Autodesk Fusion 360 part; units mm, degrees
note: some values were not read from the file. Set by a fixed rule: which sketch regions a step uses.
(part 47 of 59)
  spline S2 degree 5 poles (-27.3251, 22.3472) (-27.3252, 22.3472) (-27.3254, 22.3473) (-27.3257, 22.3474) (-27.3262, 22.3475) (-27.3269, 22.3478) (-27.3277, 22.3481) (-27.3286, 22.3484) (-27.3296, 22.3487) (-27.3308, 22.3491) (-27.332, 22.3495) (-27.3334, 22.35) (-27.3348, 22.3505) (-27.3364, 22.351) (-27.338, 22.3515) (-27.3398, 22.3521) (-27.3416, 22.3527) (-27.3435, 22.3533) (-27.3456, 22.3539) (-27.3477, 22.3546) (-27.3499, 22.3553) (-27.3523, 22.356) (-27.3547, 22.3568) (-27.3572, 22.3575) (-27.3598, 22.3583) (-27.3625, 22.3591) (-27.3652, 22.36) (-27.3681, 22.3608) (-27.371, 22.3617) (-27.3741, 22.3626) (-27.3772, 22.3635) (-27.3804, 22.3645) (-27.3837, 22.3654) (-27.387, 22.3664) (-27.3905, 22.3674) (-27.394, 22.3684) (-27.3976, 22.3694) (-27.4013, 22.3704) (-27.4051, 22.3715) (-27.409, 22.3725) (-27.4129, 22.3736) (-27.4169, 22.3747) (-27.421, 22.3758) (-27.4252, 22.3769) (-27.4294, 22.378) (-27.4337, 22.3792) (-27.4381, 22.3803) (-27.4426, 22.3815) (-27.4471, 22.3827) (-27.4517, 22.3838) (-27.4564, 22.385) (-27.4612, 22.3862) (-27.466, 22.3874) (-27.4709, 22.3887) (-27.4759, 22.3899) (-27.481, 22.3911) (-27.4861, 22.3924) (-27.4912, 22.3936) (-27.4965, 22.3949) (-27.5018, 22.3962) (-27.5072, 22.3974) (-27.5127, 22.3987) (-27.5182, 22.4) (-27.5238, 22.4013) (-27.5294, 22.4026) (-27.5352, 22.4039) (-27.5409, 22.4052) (-27.5468, 22.4065) (-27.5527, 22.4079) (-27.5587, 22.4092) (-27.5647, 22.4105) (-27.5709, 22.4118) (-27.577, 22.4132) (-27.5833, 22.4145) (-27.5896, 22.4158) (-27.5959, 22.4172) (-27.6023, 22.4185) (-27.6088, 22.4199) (-27.6154, 22.4212) (-27.622, 22.4225) (-27.6286, 22.4239) (-27.6353, 22.4252) (-27.6421, 22.4266) (-27.649, 22.4279) (-27.6559, 22.4293) (-27.6628, 22.4306) (-27.6698, 22.432) (-27.6769, 22.4333) (-27.6841, 22.4347) (-27.6912, 22.436) (-27.6985, 22.4374) (-27.7058, 22.4387) (-27.7132, 22.4401) (-27.7206, 22.4414) (-27.728, 22.4428) (-27.7356, 22.4441) (-27.7431, 22.4454) (-27.7508, 22.4468) (-27.7585, 22.4481) (-27.7662, 22.4494) (-27.774, 22.4508) (-27.7819, 22.4521) (-27.7898, 22.4534) (-27.7977, 22.4547) (-27.8057, 22.456) (-27.8138, 22.4573) (-27.8219, 22.4586) (-27.8301, 22.4599) (-27.8383, 22.4612) (-27.8466, 22.4625) (-27.8549, 22.4638) (-27.8633, 22.4651) (-27.8717, 22.4664) (-27.8802, 22.4676) (-27.8887, 22.4689) (-27.8973, 22.4701) (-27.9059, 22.4714) (-27.9146, 22.4726) (-27.9233, 22.4739) (-27.9321, 22.4751) (-27.9409, 22.4763) (-27.9498, 22.4776) (-27.9587, 22.4788) (-27.9677, 22.48) (-27.9767, 22.4812) (-27.9858, 22.4824) (-27.9949, 22.4836) (-28.004, 22.4847) (-28.0133, 22.4859) (-28.0225, 22.4871) (-28.0318, 22.4882) (-28.0412, 22.4894) (-28.0506, 22.4905) (-28.06, 22.4916) (-28.0695, 22.4928) (-28.079, 22.4939) (-28.0886, 22.495) (-28.0982, 22.4961) (-28.1079, 22.4972) (-28.1176, 22.4983) (-28.1274, 22.4993) (-28.1372, 22.5004) (-28.147, 22.5014) (-28.1569, 22.5025) (-28.1668, 22.5035) (-28.1768, 22.5045) (-28.1868, 22.5055) (-28.1969, 22.5065) (-28.207, 22.5075) (-28.2172, 22.5085) (-28.2274, 22.5095) (-28.2376, 22.5104) (-28.2479, 22.5114) (-28.2582, 22.5123) (-28.2686, 22.5133) (-28.279, 22.5142) (-28.2894, 22.5151) (-28.2999, 22.516) (-28.3105, 22.5169) (-28.321, 22.5177) (-28.3317, 22.5186) (-28.3423, 22.5195) (-28.353, 22.5203) (-28.3638, 22.5211) (-28.3745, 22.5219) (-28.3854, 22.5227) (-28.3962, 22.5235) (-28.4071, 22.5243) (-28.4181, 22.5251) (-28.429, 22.5258) (-28.44, 22.5266) (-28.4511, 22.5273) (-28.4622, 22.528) (-28.4733, 22.5287) (-28.4845, 22.5294) (-28.4957, 22.5301) (-28.507, 22.5308) (-28.5183, 22.5314) (-28.5296, 22.5321) (-28.541, 22.5327) (-28.5524, 22.5333) (-28.5638, 22.5339) (-28.5753, 22.5345) (-28.5868, 22.5351) (-28.5984, 22.5356) (-28.61, 22.5362) (-28.6216, 22.5367) (-28.6333, 22.5372) (-28.645, 22.5377) (-28.6567, 22.5382) (-28.6685, 22.5387) (-28.6803, 22.5392) (-28.6922, 22.5396) (-28.7041, 22.54) (-28.716, 22.5405) (-28.728, 22.5409) (-28.74, 22.5412) (-28.752, 22.5416) (-28.7641, 22.542) (-28.7762, 22.5423) (-28.7883, 22.5427) (-28.8005, 22.543) (-28.8127, 22.5433) (-28.8249, 22.5436) (-28.8372, 22.5438) (-28.8495, 22.5441) (-28.8619, 22.5443) (-28.8743, 22.5445) (-28.8867, 22.5448) (-28.8991, 22.5449) (-28.9116, 22.5451) (-28.9241, 22.5453) (-28.9367, 22.5454) (-28.9493, 22.5456) (-28.9619, 22.5457) (-28.9745, 22.5458) (-28.9872, 22.5458) (-29, 22.5459) (-29.0127, 22.546) (-29.0255, 22.546) (-29.0383, 22.546) (-29.0512, 22.546) (-29.0641, 22.546) (-29.077, 22.546) (-29.0899, 22.5459) (-29.1029, 22.5458) (-29.1159, 22.5458) (-29.129, 22.5457) (-29.142, 22.5455) (-29.1551, 22.5454) (-29.1683, 22.5453) (-29.1815, 22.5451) (-29.1947, 22.5449) (-29.2079, 22.5447) (-29.2212, 22.5445) (-29.2345, 22.5442) (-29.2478, 22.544) (-29.2612, 22.5437) (-29.2745, 22.5434) (-29.288, 22.5431) (-29.3014, 22.5428) (-29.3122, 22.5425) (-29.3203, 22.5423) (-29.3257, 22.5422) (-29.3284, 22.5421) knots 0 0 0 0 0 0 0.00416667 0.00833333 0.0125 0.01666667 0.02083333 0.025 0.02916667 0.03333333 0.0375 0.04166667 0.04583333 0.05 0.05416667 0.05833333 0.0625 0.06666667 0.07083333 0.075 0.07916667 0.08333333 0.0875 0.09166667 0.09583333 0.1 0.10416667 0.10833333 0.1125 0.11666667 0.12083333 0.125 0.12916667 0.13333333 0.1375 0.14166667 0.14583333 0.15 0.15416667 0.15833333 0.1625 0.16666667 0.17083333 0.175 0.17916667 0.18333333 0.1875 0.19166667 0.19583333 0.2 0.20416667 0.20833333 0.2125 0.21666667 0.22083333 0.225 0.22916667 0.23333333 0.2375 0.24166667 0.24583333 0.25 0.25416667 0.25833333 0.2625 0.26666667 0.27083333 0.275 0.27916667 0.28333333 0.2875 0.29166667 0.29583333 0.3 0.30416667 0.30833333 0.3125 0.31666667 0.32083333 0.325 0.32916667 0.33333333 0.3375 0.34166667 0.34583333 0.35 0.35416667 0.35833333 0.3625 0.36666667 0.37083333 0.375 0.37916667 0.38333333 0.3875 0.39166667 0.39583333 0.4 0.40416667 0.40833333 0.4125 0.41666667 0.42083333 0.425 0.42916667 0.43333333 0.4375 0.44166667 0.44583333 0.45 0.45416667 0.45833333 0.4625 0.46666667 0.47083333 0.475 0.47916667 0.48333333 0.4875 0.49166667 0.49583333 0.5 0.50416667 0.50833333 0.5125 0.51666667 0.52083333 0.525 0.52916667 0.53333333 0.5375 0.54166667 0.54583333 0.55 0.55416667 0.55833333 0.5625 0.56666667 0.57083333 0.575 0.57916667 0.58333333 0.5875 0.59166667 0.59583333 0.6 0.60416667 0.60833333 0.6125 0.61666667 0.62083333 0.625 0.62916667 0.63333333 0.6375 0.64166667 0.64583333 0.65 0.65416667 0.65833333 0.6625 0.66666667 0.67083333 0.675 0.67916667 0.68333333 0.6875 0.69166667 0.69583333 0.7 0.70416667 0.70833333 0.7125 0.71666667 0.72083333 0.725 0.72916667 0.73333333 0.7375 0.74166667 0.74583333 0.75 0.75416667 0.75833333 0.7625 0.76666667 0.77083333 0.775 0.77916667 0.78333333 0.7875 0.79166667 0.79583333 0.8 0.80416667 0.80833333 0.8125 0.81666667 0.82083333 0.825 0.82916667 0.83333333 0.8375 0.84166667 0.84583333 0.85 0.85416667 0.85833333 0.8625 0.86666667 0.87083333 0.875 0.87916667 0.88333333 0.8875 0.89166667 0.89583333 0.9 0.90416667 0.90833333 0.9125 0.91666667 0.92083333 0.925 0.92916667 0.93333333 0.9375 0.94166667 0.94583333 0.95 0.95416667 0.95833333 0.9625 0.96666667 0.97083333 0.975 0.97916667 0.98333333 0.9875 0.99166667 0.99583333 1 1 1 1 1 1
  arc A3 (-29.3284, 22.5421) -> (-29.6298, 21.6146) centre (0, 12.5) ccw
  spline S3 degree 5 poles (-29.6298, 21.6146) (-29.6276, 21.6129) (-29.6234, 21.6096) (-29.6169, 21.6047) (-29.6084, 21.5981) (-29.5977, 21.59) (-29.587, 21.5818) (-29.5763, 21.5737) (-29.5657, 21.5657) (-29.555, 21.5576) (-29.5444, 21.5496) (-29.5338, 21.5416) (-29.5232, 21.5337) (-29.5127, 21.5258) (-29.5021, 21.5179) (-29.4915, 21.5101) (-29.481, 21.5022) (-29.4705, 21.4945) (-29.46, 21.4867) (-29.4495, 21.479) (-29.4391, 21.4713) (-29.4286, 21.4637) (-29.4182, 21.456) (-29.4078, 21.4485) (-29.3974, 21.4409) (-29.387, 21.4334) (-29.3766, 21.4259) (-29.3663, 21.4184) (-29.356, 21.411) (-29.3457, 21.4036) (-29.3354, 21.3963) (-29.3251, 21.3889) (-29.3148, 21.3816) (-29.3046, 21.3744) (-29.2944, 21.3671) (-29.2842, 21.36) (-29.274, 21.3528) (-29.2638, 21.3457) (-29.2537, 21.3386) (-29.2435, 21.3315) (-29.2334, 21.3245) (-29.2233, 21.3175) (-29.2132, 21.3105) (-29.2032, 21.3036) (-29.1932, 21.2967) (-29.1831, 21.2898) (-29.1731, 21.283) (-29.1632, 21.2762) (-29.1532, 21.2694) (-29.1433, 21.2626) (-29.1334, 21.2559) (-29.1235, 21.2493) (-29.1136, 21.2426) (-29.1037, 21.236) (-29.0939, 21.2295) (-29.0841, 21.2229) (-29.0743, 21.2164) (-29.0646, 21.2099) (-29.0548, 21.2035) (-29.0451, 21.1971) (-29.0354, 21.1907) (-29.0257, 21.1844) (-29.016, 21.1781) (-29.0064, 21.1718) (-28.9968, 21.1656) (-28.9872, 21.1593) (-28.9776, 21.1532) (-28.9681, 21.147) (-28.9586, 21.1409) (-28.9491, 21.1348) (-28.9396, 21.1288) (-28.9302, 21.1228) (-28.9207, 21.1168) (-28.9113, 21.1109) (-28.902, 21.105) (-28.8926, 21.0991) (-28.8833, 21.0932) (-28.874, 21.0874) (-28.8647, 21.0817) (-28.8555, 21.0759) (-28.8462, 21.0702) (-28.837, 21.0645) (-28.8279, 21.0589) (-28.8187, 21.0533) (-28.8096, 21.0477) (-28.8005, 21.0422) (-28.7914, 21.0367) (-28.7824, 21.0312) (-28.7734, 21.0257) (-28.7644, 21.0203) (-28.7554, 21.015) (-28.7465, 21.0096) (-28.7376, 21.0043) (-28.7287, 20.999) (-28.7199, 20.9938) (-28.711, 20.9886) (-28.7022, 20.9834) (-28.6935, 20.9783) (-28.6847, 20.9732) (-28.676, 20.9681) (-28.6674, 20.963) (-28.6587, 20.958) (-28.6501, 20.9531) (-28.6415, 20.9481) (-28.633, 20.9432) (-28.6244, 20.9384) (-28.616, 20.9335) (-28.6075, 20.9287) (-28.5991, 20.9239) (-28.5907, 20.9192) (-28.5823, 20.9145) (-28.574, 20.9098) (-28.5657, 20.9052) (-28.5574, 20.9006) (-28.5491, 20.896) (-28.5409, 20.8915) (-28.5328, 20.887) (-28.5246, 20.8825) (-28.5165, 20.8781) (-28.5085, 20.8737) (-28.5004, 20.8693) (-28.4924, 20.865) (-28.4845, 20.8607) (-28.4765, 20.8565) (-28.4686, 20.8522) (-28.4608, 20.848) (-28.4529, 20.8439) (-28.4452, 20.8398) (-28.4374, 20.8357) (-28.4297, 20.8316) (-28.422, 20.8276) (-28.4144, 20.8236) (-28.4068, 20.8196) (-28.3992, 20.8157) (-28.3917, 20.8118) (-28.3842, 20.808) (-28.3767, 20.8042) (-28.3693, 20.8004) (-28.3619, 20.7966) (-28.3546, 20.7929) (-28.3473, 20.7892) (-28.3401, 20.7856) (-28.3329, 20.782) (-28.3257, 20.7784) (-28.3186, 20.7748) (-28.3115, 20.7713) (-28.3044, 20.7678) (-28.2974, 20.7644) (-28.2905, 20.761) (-28.2835, 20.7576) (-28.2767, 20.7543) (-28.2698, 20.751) (-28.263, 20.7477) (-28.2563, 20.7445) (-28.2496, 20.7412) (-28.2429, 20.7381) (-28.2363, 20.7349) (-28.2298, 20.7318) (-28.2233, 20.7288) (-28.2168, 20.7257) (-28.2104, 20.7227) (-28.204, 20.7198) (-28.1977, 20.7169) (-28.1914, 20.714) (-28.1851, 20.7111) (-28.179, 20.7083) (-28.1728, 20.7055) (-28.1667, 20.7027) (-28.1607, 20.7) (-28.1547, 20.6973) (-28.1488, 20.6947) (-28.1429, 20.692) (-28.1371, 20.6895) (-28.1313, 20.6869) (-28.1256, 20.6844) (-28.1199, 20.6819) (-28.1143, 20.6795) (-28.1087, 20.677) (-28.1032, 20.6747) (-28.0978, 20.6723) (-28.0924, 20.67) (-28.087, 20.6677) (-28.0818, 20.6655) (-28.0765, 20.6633) (-28.0714, 20.6611) (-28.0663, 20.659) (-28.0612, 20.6569) (-28.0562, 20.6548) (-28.0513, 20.6528) (-28.0464, 20.6508) (-28.0416, 20.6488) (-28.0369, 20.6469) (-28.0322, 20.645) (-28.0276, 20.6432) (-28.023, 20.6413) (-28.0185, 20.6395) (-28.0141, 20.6378) (-28.0097, 20.6361) (-28.0054, 20.6344) (-28.0012, 20.6327) (-27.997, 20.6311) (-27.9929, 20.6295) (-27.9889, 20.628) (-27.9849, 20.6265) (-27.9811, 20.625) (-27.9772, 20.6236) (-27.9735, 20.6222) (-27.9698, 20.6208) (-27.9662, 20.6194) (-27.9627, 20.6181) (-27.9593, 20.6169) (-27.9559, 20.6156) (-27.9526, 20.6144) (-27.9494, 20.6133) (-27.9462, 20.6121) (-27.9432, 20.6111) (-27.9402, 20.61) (-27.9373, 20.609) (-27.9345, 20.608) (-27.9318, 20.607) (-27.9291, 20.6061) (-27.9265, 20.6052) (-27.9241, 20.6044) (-27.9217, 20.6036) (-27.9194, 20.6028) (-27.9172, 20.602) (-27.915, 20.6013) (-27.913, 20.6007) (-27.9111, 20.6) (-27.9092, 20.5994) (-27.9075, 20.5988) (-27.9058, 20.5983) (-27.9043, 20.5978) (-27.9028, 20.5973) (-27.9015, 20.5969) (-27.9002, 20.5965) (-27.8991, 20.5962) (-27.898, 20.5958) (-27.8971, 20.5956) (-27.8963, 20.5953) (-27.8956, 20.5951) (-27.8951, 20.5949) (-27.8948, 20.5948) (-27.8946, 20.5948) (-27.8945, 20.5948) knots -1 -1 -1 -1 -1 -1 -0.99583333 -0.99166667 -0.9875 -0.98333333 -0.97916667 -0.975 -0.97083333 -0.96666667 -0.9625 -0.95833333 -0.95416667 -0.95 -0.94583333 -0.94166667 -0.9375 -0.93333333 -0.92916667 -0.925 -0.92083333 -0.91666667 -0.9125 -0.90833333 -0.90416667 -0.9 -0.89583333 -0.89166667 -0.8875 -0.88333333 -0.87916667 -0.875 -0.87083333 -0.86666667 -0.8625 -0.85833333 -0.85416667 -0.85 -0.84583333 -0.84166667 -0.8375 -0.83333333 -0.82916667 -0.825 -0.82083333 -0.81666667 -0.8125 -0.80833333 -0.80416667 -0.8 -0.79583333 -0.79166667 -0.7875 -0.78333333 -0.77916667 -0.775 -0.77083333 -0.76666667 -0.7625 -0.75833333 -0.75416667 -0.75 -0.74583333 -0.74166667 -0.7375 -0.73333333 -0.72916667 -0.725 -0.72083333 -0.71666667 -0.7125 -0.70833333 -0.70416667 -0.7 -0.69583333 -0.69166667 -0.6875 -0.68333333 -0.67916667 -0.675 -0.67083333 -0.66666667 -0.6625 -0.65833333 -0.65416667 -0.65 -0.64583333 -0.64166667 -0.6375 -0.63333333 -0.62916667 -0.625 -0.62083333 -0.61666667 -0.6125 -0.60833333 -0.60416667 -0.6 -0.59583333 -0.59166667 -0.5875 -0.58333333 -0.57916667 -0.575 -0.57083333 -0.56666667 -0.5625 -0.55833333 -0.55416667 -0.55 -0.54583333 -0.54166667 -0.5375 -0.53333333 -0.52916667 -0.525 -0.52083333 -0.51666667 -0.5125 -0.50833333 -0.50416667 -0.5 -0.49583333 -0.49166667 -0.4875 -0.48333333 -0.47916667 -0.475 -0.47083333 -0.46666667 -0.4625 -0.45833333 -0.45416667 -0.45 -0.44583333 -0.44166667 -0.4375 -0.43333333 -0.42916667 -0.425 -0.42083333 -0.41666667 -0.4125 -0.40833333 -0.40416667 -0.4 -0.39583333 -0.39166667 -0.3875 -0.38333333 -0.37916667 -0.375 -0.37083333 -0.36666667 -0.3625 -0.35833333 -0.35416667 -0.35 -0.34583333 -0.34166667 -0.3375 -0.33333333 -0.32916667 -0.325 -0.32083333 -0.31666667 -0.3125 -0.30833333 -0.30416667 -0.3 -0.29583333 -0.29166667 -0.2875 -0.28333333 -0.27916667 -0.275 -0.27083333 -0.26666667 -0.2625 -0.25833333 -0.25416667 -0.25 -0.24583333 -0.24166667 -0.2375 -0.23333333 -0.22916667 -0.225 -0.22083333 -0.21666667 -0.2125 -0.20833333 -0.20416667 -0.2 -0.19583333 -0.19166667 -0.1875 -0.18333333 -0.17916667 -0.175 -0.17083333 -0.16666667 -0.1625 -0.15833333 -0.15416667 -0.15 -0.14583333 -0.14166667 -0.1375 -0.13333333 -0.12916667 -0.125 -0.12083333 -0.11666667 -0.1125 -0.10833333 -0.10416667 -0.1 -0.09583333 -0.09166667 -0.0875 -0.08333333 -0.07916667 -0.075 -0.07083333 -0.06666667 -0.0625 -0.05833333 -0.05416667 -0.05 -0.04583333 -0.04166667 -0.0375 -0.03333333 -0.02916667 -0.025 -0.02083333 -0.01666667 -0.0125 -0.00833333 -0.00416667 0 0 0 0 0 0
  line L7 (-27.8945, 20.5948) -> (-27.8937, 20.5945)
  line L8 (-27.8937, 20.5945) -> (-27.6109, 20.5125)
  arc A4 (-27.6109, 20.5125) -> (-27.918, 19.3665) centre (0, 12.5) ccw
  line L9 (-27.918, 19.3665) -> (-28.2039, 19.4368)
  line L10 (-28.2039, 19.4368) -> (-28.2047, 19.437)
  spline S4 degree 5 poles (-28.2047, 19.437) (-28.2048, 19.437) (-28.205, 19.437) (-28.2053, 19.4371) (-28.2058, 19.4372) (-28.2065, 19.4374) (-28.2074, 19.4376) (-28.2083, 19.4378) (-28.2094, 19.4381) (-28.2106, 19.4383) (-28.2118, 19.4386) (-28.2132, 19.4389) (-28.2147, 19.4392) (-28.2163, 19.4396) (-28.218, 19.4399) (-28.2198, 19.4403) (-28.2217, 19.4407) (-28.2237, 19.4411) (-28.2258, 19.4416) (-28.228, 19.442) (-28.2303, 19.4425) (-28.2327, 19.4429) (-28.2351, 19.4434) (-28.2377, 19.4439) (-28.2404, 19.4445) (-28.2431, 19.445) (-28.246, 19.4455) (-28.2489, 19.4461) (-28.2519, 19.4466) (-28.255, 19.4472) (-28.2582, 19.4478) (-28.2615, 19.4484) (-28.2649, 19.449) (-28.2683, 19.4496) (-28.2719, 19.4502) (-28.2755, 19.4508) (-28.2792, 19.4515) (-28.283, 19.4521) (-28.2868, 19.4528) (-28.2908, 19.4534) (-28.2948, 19.4541) (-28.2989, 19.4547) (-28.3031, 19.4554) (-28.3074, 19.4561) (-28.3117, 19.4568) (-28.3161, 19.4574) (-28.3206, 19.4581) (-28.3252, 19.4588) (-28.3298, 19.4595) (-28.3345, 19.4602) (-28.3393, 19.4609) (-28.3442, 19.4616) (-28.3491, 19.4623) (-28.3541, 19.463) (-28.3592, 19.4637) (-28.3643, 19.4644) (-28.3695, 19.4651) (-28.3748, 19.4658) (-28.3802, 19.4665) (-28.3856, 19.4672) (-28.3911, 19.4679) (-28.3966, 19.4686) (-28.4023, 19.4693) (-28.408, 19.47) (-28.4137, 19.4707) (-28.4196, 19.4714) (-28.4255, 19.4721) (-28.4314, 19.4728) (-28.4374, 19.4735) (-28.4435, 19.4742) (-28.4497, 19.4749) (-28.4559, 19.4756) (-28.4622, 19.4763) (-28.4685, 19.4769) (-28.4749, 19.4776) (-28.4814, 19.4783) (-28.4879, 19.4789) (-28.4945, 19.4796) (-28.5011, 19.4803) (-28.5078, 19.4809) (-28.5146, 19.4816) (-28.5214, 19.4822) (-28.5283, 19.4828) (-28.5353, 19.4835) (-28.5423, 19.4841) (-28.5493, 19.4847) (-28.5564, 19.4853) (-28.5636, 19.4859) (-28.5709, 19.4865) (-28.5781, 19.4871) (-28.5855, 19.4877) (-28.5929, 19.4882) (-28.6004, 19.4888) (-28.6079, 19.4894) (-28.6154, 19.4899) (-28.6231, 19.4905) (-28.6307, 19.491) (-28.6385, 19.4915) (-28.6463, 19.4921) (-28.6541, 19.4926) (-28.662, 19.4931) (-28.67, 19.4936) (-28.678, 19.494) (-28.686, 19.4945) (-28.6941, 19.495) (-28.7023, 19.4954) (-28.7105, 19.4959) (-28.7187, 19.4963) (-28.727, 19.4968) (-28.7354, 19.4972) (-28.7438, 19.4976) (-28.7523, 19.498) (-28.7608, 19.4984) (-28.7694, 19.4987) (-28.778, 19.4991) (-28.7866, 19.4995) (-28.7953, 19.4998) (-28.8041, 19.5001) (-28.8129, 19.5005) (-28.8218, 19.5008) (-28.8307, 19.5011) (-28.8396, 19.5014) (-28.8486, 19.5016) (-28.8577, 19.5019) (-28.8668, 19.5021) (-28.8759, 19.5024) (-28.8851, 19.5026) (-28.8943, 19.5028) (-28.9036, 19.503) (-28.9129, 19.5032) (-28.9223, 19.5034) (-28.9317, 19.5036) (-28.9412, 19.5037) (-28.9507, 19.5038) (-28.9602, 19.504) (-28.9698, 19.5041) (-28.9795, 19.5042) (-28.9892, 19.5043) (-28.9989, 19.5043) (-29.0087, 19.5044) (-29.0185, 19.5044) (-29.0284, 19.5045) (-29.0383, 19.5045) (-29.0482, 19.5045) (-29.0582, 19.5045) (-29.0682, 19.5044) (-29.0783, 19.5044) (-29.0884, 19.5043) (-29.0986, 19.5043) (-29.1088, 19.5042) (-29.119, 19.5041) (-29.1293, 19.504) (-29.1396, 19.5038) (-29.15, 19.5037) (-29.1604, 19.5035) (-29.1708, 19.5034) (-29.1813, 19.5032) (-29.1919, 19.503) (-29.2024, 19.5028) (-29.213, 19.5025) (-29.2237, 19.5023) (-29.2344, 19.502) (-29.2451, 19.5017) (-29.2559, 19.5014) (-29.2667, 19.5011) (-29.2775, 19.5008) (-29.2884, 19.5004) (-29.2993, 19.5001) (-29.3103, 19.4997) (-29.3213, 19.4993) (-29.3323, 19.4989) (-29.3434, 19.4984) (-29.3545, 19.498) (-29.3657, 19.4975) (-29.3768, 19.497) (-29.3881, 19.4965) (-29.3993, 19.496) (-29.4106, 19.4955) (-29.422, 19.495) (-29.4333, 19.4944) (-29.4447, 19.4938) (-29.4562, 19.4932) (-29.4677, 19.4926) (-29.4792, 19.492) (-29.4907, 19.4913) (-29.5023, 19.4906) (-29.514, 19.49) (-29.5256, 19.4892) (-29.5373, 19.4885) (-29.549, 19.4878) (-29.5608, 19.487) (-29.5726, 19.4863) (-29.5844, 19.4855) (-29.5963, 19.4846) (-29.6082, 19.4838) (-29.6201, 19.483) (-29.6321, 19.4821) (-29.6441, 19.4812) (-29.6562, 19.4803) (-29.6682, 19.4794) (-29.6803, 19.4784) (-29.6925, 19.4775) (-29.7047, 19.4765) (-29.7169, 19.4755) (-29.7291, 19.4745) (-29.7414, 19.4735) (-29.7537, 19.4724) (-29.766, 19.4713) (-29.7784, 19.4702) (-29.7908, 19.4691) (-29.8032, 19.468) (-29.8157, 19.4669) (-29.8282, 19.4657) (-29.8407, 19.4645) (-29.8533, 19.4633) (-29.8659, 19.4621) (-29.8785, 19.4608) (-29.8912, 19.4596) (-29.9039, 19.4583) (-29.9166, 19.457) (-29.9293, 19.4556) (-29.9421, 19.4543) (-29.9549, 19.4529) (-29.9678, 19.4516) (-29.9806, 19.4501) (-29.9935, 19.4487) (-30.0065, 19.4473) (-30.0194, 19.4458) (-30.0324, 19.4443) (-30.0455, 19.4428) (-30.0585, 19.4413) (-30.0716, 19.4398) (-30.0847, 19.4382) (-30.0979, 19.4366) (-30.111, 19.435) (-30.1242, 19.4334) (-30.1375, 19.4317) (-30.1507, 19.4301) (-30.164, 19.4284) (-30.1773, 19.4267) (-30.1907, 19.425) (-30.2014, 19.4236) (-30.2094, 19.4225) (-30.2148, 19.4218) (-30.2174, 19.4214) knots 0 0 0 0 0 0 0.00416667 0.00833333 0.0125 0.01666667 0.02083333 0.025 0.02916667 0.03333333 0.0375 0.04166667 0.04583333 0.05 0.05416667 0.05833333 0.0625 0.06666667 0.07083333 0.075 0.07916667 0.08333333 0.0875 0.09166667 0.09583333 0.1 0.10416667 0.10833333 0.1125 0.11666667 0.12083333 0.125 0.12916667 0.13333333 0.1375 0.14166667 0.14583333 0.15 0.15416667 0.15833333 0.1625 0.16666667 0.17083333 0.175 0.17916667 0.18333333 0.1875 0.19166667 0.19583333 0.2 0.20416667 0.20833333 0.2125 0.21666667 0.22083333 0.225 0.22916667 0.23333333 0.2375 0.24166667 0.24583333 0.25 0.25416667 0.25833333 0.2625 0.26666667 0.27083333 0.275 0.27916667 0.28333333 0.2875 0.29166667 0.29583333 0.3 0.30416667 0.30833333 0.3125 0.31666667 0.32083333 0.325 0.32916667 0.33333333 0.3375 0.34166667 0.34583333 0.35 0.35416667 0.35833333 0.3625 0.36666667 0.37083333 0.375 0.37916667 0.38333333 0.3875 0.39166667 0.39583333 0.4 0.40416667 0.40833333 0.4125 0.41666667 0.42083333 0.425 0.42916667 0.43333333 0.4375 0.44166667 0.44583333 0.45 0.45416667 0.45833333 0.4625 0.46666667 0.47083333 0.475 0.47916667 0.48333333 0.4875 0.49166667 0.49583333 0.5 0.50416667 0.50833333 0.5125 0.51666667 0.52083333 0.525 0.52916667 0.53333333 0.5375 0.54166667 0.54583333 0.55 0.55416667 0.55833333 0.5625 0.56666667 0.57083333 0.575 0.57916667 0.58333333 0.5875 0.59166667 0.59583333 0.6 0.60416667 0.60833333 0.6125 0.61666667 0.62083333 0.625 0.62916667 0.63333333 0.6375 0.64166667 0.64583333 0.65 0.65416667 0.65833333 0.6625 0.66666667 0.67083333 0.675 0.67916667 0.68333333 0.6875 0.69166667 0.69583333 0.7 0.70416667 0.70833333 0.7125 0.71666667 0.72083333 0.725 0.72916667 0.73333333 0.7375 0.74166667 0.74583333 0.75 0.75416667 0.75833333 0.7625 0.76666667 0.77083333 0.775 0.77916667 0.78333333 0.7875 0.79166667 0.79583333 0.8 0.80416667 0.80833333 0.8125 0.81666667 0.82083333 0.825 0.82916667 0.83333333 0.8375 0.84166667 0.84583333 0.85 0.85416667 0.85833333 0.8625 0.86666667 0.87083333 0.875 0.87916667 0.88333333 0.8875 0.89166667 0.89583333 0.9 0.90416667 0.90833333 0.9125 0.91666667 0.92083333 0.925 0.92916667 0.93333333 0.9375 0.94166667 0.94583333 0.95 0.95416667 0.95833333 0.9625 0.96666667 0.97083333 0.975 0.97916667 0.98333333 0.9875 0.99166667 0.99583333 1 1 1 1 1 1
  arc A5 (-30.2174, 19.4214) -> (-30.4202, 18.4675) centre (0, 12.5) ccw
  spline S5 degree 5 poles (-30.4202, 18.4675) (-30.4179, 18.4661) (-30.4133, 18.4633) (-30.4064, 18.459) (-30.3972, 18.4534) (-30.3857, 18.4464) (-30.3742, 18.4394) (-30.3628, 18.4325) (-30.3513, 18.4255) (-30.3399, 18.4187) (-30.3285, 18.4118) (-30.3171, 18.405) (-30.3058, 18.3982) (-30.2944, 18.3914) (-30.2831, 18.3847) (-30.2718, 18.378) (-30.2605, 18.3713) (-30.2492, 18.3647) (-30.238, 18.3581) (-30.2268, 18.3515) (-30.2156, 18.3449) (-30.2044, 18.3384) (-30.1932, 18.3319) (-30.1821, 18.3255) (-30.1709, 18.3191) (-30.1598, 18.3127) (-30.1487, 18.3063) (-30.1377, 18.3) (-30.1266, 18.2937) (-30.1156, 18.2874) (-30.1046, 18.2811) (-30.0936, 18.2749) (-30.0826, 18.2688) (-30.0717, 18.2626) (-30.0608, 18.2565) (-30.0499, 18.2504) (-30.039, 18.2443) (-30.0281, 18.2383) (-30.0173, 18.2323) (-30.0065, 18.2263) (-29.9957, 18.2204) (-29.9849, 18.2145) (-29.9742, 18.2086) (-29.9634, 18.2028) (-29.9527, 18.197) (-29.9421, 18.1912) (-29.9314, 18.1854) (-29.9208, 18.1797) (-29.9102, 18.174) (-29.8996, 18.1683) (-29.889, 18.1627) (-29.8785, 18.1571) (-29.868, 18.1515) (-29.8575, 18.146) (-29.847, 18.1405) (-29.8366, 18.135) (-29.8262, 18.1296) (-29.8158, 18.1242) (-29.8054, 18.1188) (-29.7951, 18.1134) (-29.7847, 18.1081) (-29.7745, 18.1028) (-29.7642, 18.0975) (-29.754, 18.0923) (-29.7437, 18.0871) (-29.7336, 18.0819) (-29.7234, 18.0768) (-29.7133, 18.0717) (-29.7032, 18.0666) (-29.6931, 18.0615) (-29.683, 18.0565) (-29.673, 18.0515) (-29.663, 18.0466) (-29.653, 18.0416) (-29.6431, 18.0367) (-29.6332, 18.0319) (-29.6233, 18.027) (-29.6134, 18.0222) (-29.6036, 18.0175) (-29.5938, 18.0127) (-29.584, 18.008) (-29.5743, 18.0033) (-29.5646, 17.9987) (-29.5549, 17.994) (-29.5452, 17.9895) (-29.5356, 17.9849) (-29.526, 17.9804) (-29.5165, 17.9759) (-29.5069, 17.9714) (-29.4974, 17.967) (-29.4879, 17.9625) (-29.4785, 17.9582) (-29.4691, 17.9538) (-29.4597, 17.9495) (-29.4504, 17.9452) (-29.441, 17.941) (-29.4318, 17.9367) (-29.4225, 17.9325) (-29.4133, 17.9284) (-29.4041, 17.9242) (-29.395, 17.9201) (-29.3858, 17.9161) (-29.3767, 17.912) (-29.3677, 17.908) (-29.3587, 17.904) (-29.3497, 17.9001) (-29.3407, 17.8961) (-29.3318, 17.8922) (-29.3229, 17.8884) (-29.3141, 17.8846) (-29.3053, 17.8807) (-29.2965, 17.877) (-29.2878, 17.8732) (-29.279, 17.8695) (-29.2704, 17.8658) (-29.2617, 17.8622) (-29.2531, 17.8586) (-29.2446, 17.855) (-29.2361, 17.8514) (-29.2276, 17.8479) (-29.2191, 17.8444) (-29.2107, 17.8409) (-29.2023, 17.8375) (-29.194, 17.8341) (-29.1857, 17.8307) (-29.1775, 17.8273) (-29.1692, 17.824) (-29.1611, 17.8207) (-29.1529, 17.8175) (-29.1448, 17.8143) (-29.1368, 17.8111) (-29.1288, 17.8079) (-29.1208, 17.8047) (-29.1129, 17.8016) (-29.105, 17.7986) (-29.0971, 17.7955) (-29.0893, 17.7925) (-29.0815, 17.7895) (-29.0738, 17.7865) (-29.0661, 17.7836) (-29.0585, 17.7807) (-29.0509, 17.7778) (-29.0433, 17.775) (-29.0358, 17.7722) (-29.0284, 17.7694) (-29.021, 17.7666) (-29.0136, 17.7639) (-29.0063, 17.7612) (-28.999, 17.7586) (-28.9918, 17.7559) (-28.9846, 17.7533) (-28.9774, 17.7508) (-28.9703, 17.7482) (-28.9633, 17.7457) (-28.9563, 17.7432) (-28.9493, 17.7408) (-28.9424, 17.7383) (-28.9356, 17.7359) (-28.9288, 17.7336) (-28.922, 17.7312) (-28.9153, 17.7289) (-28.9087, 17.7266) (-28.9021, 17.7244) (-28.8955, 17.7222) (-28.889, 17.72) (-28.8826, 17.7178) (-28.8762, 17.7157) (-28.8699, 17.7136) (-28.8636, 17.7115) (-28.8573, 17.7094) (-28.8512, 17.7074) (-28.8451, 17.7054) (-28.839, 17.7035) (-28.833, 17.7015) (-28.827, 17.6996) (-28.8211, 17.6978) (-28.8153, 17.6959) (-28.8095, 17.6941) (-28.8038, 17.6923) (-28.7981, 17.6905) (-28.7925, 17.6888) (-28.7869, 17.6871) (-28.7815, 17.6854) (-28.776, 17.6838) (-28.7707, 17.6822) (-28.7654, 17.6806) (-28.7601, 17.679) (-28.7549, 17.6775) (-28.7498, 17.676) (-28.7448, 17.6745) (-28.7398, 17.673) (-28.7349, 17.6716) (-28.73, 17.6702) (-28.7252, 17.6689) (-28.7205, 17.6675) (-28.7158, 17.6662) (-28.7112, 17.6649) (-28.7067, 17.6637) (-28.7023, 17.6625) (-28.6979, 17.6613) (-28.6936, 17.6601) (-28.6893, 17.6589) (-28.6852, 17.6578) (-28.6811, 17.6567) (-28.6771, 17.6557) (-28.6731, 17.6546) (-28.6693, 17.6536) (-28.6655, 17.6527) (-28.6617, 17.6517) (-28.6581, 17.6508) (-28.6545, 17.6499) (-28.6511, 17.649) (-28.6477, 17.6481) (-28.6443, 17.6473) (-28.6411, 17.6465) (-28.6379, 17.6458) (-28.6349, 17.645) (-28.6319, 17.6443) (-28.629, 17.6436) (-28.6262, 17.643) (-28.6234, 17.6423) (-28.6208, 17.6417) (-28.6182, 17.6411) (-28.6158, 17.6406) (-28.6134, 17.64) (-28.6111, 17.6395) (-28.6089, 17.639) (-28.6069, 17.6386) (-28.6049, 17.6381) (-28.603, 17.6377) (-28.6012, 17.6374) (-28.5995, 17.637) (-28.5979, 17.6367) (-28.5964, 17.6363) (-28.595, 17.6361) (-28.5937, 17.6358) (-28.5925, 17.6356) (-28.5915, 17.6354) (-28.5905, 17.6352) (-28.5896, 17.635) (-28.5889, 17.6349) (-28.5884, 17.6348) (-28.5881, 17.6347) (-28.5879, 17.6347) (-28.5878, 17.6346) knots -1 -1 -1 -1 -1 -1 -0.99583333 -0.99166667 -0.9875 -0.98333333 -0.97916667 -0.975 -0.97083333 -0.96666667 -0.9625 -0.95833333 -0.95416667 -0.95 -0.94583333 -0.94166667 -0.9375 -0.93333333 -0.92916667 -0.925 -0.92083333 -0.91666667 -0.9125 -0.90833333 -0.90416667 -0.9 -0.89583333 -0.89166667 -0.8875 -0.88333333 -0.87916667 -0.875 -0.87083333 -0.86666667 -0.8625 -0.85833333 -0.85416667 -0.85 -0.84583333 -0.84166667 -0.8375 -0.83333333 -0.82916667 -0.825 -0.82083333 -0.81666667 -0.8125 -0.80833333 -0.80416667 -0.8 -0.79583333 -0.79166667 -0.7875 -0.78333333 -0.77916667 -0.775 -0.77083333 -0.76666667 -0.7625 -0.75833333 -0.75416667 -0.75 -0.74583333 -0.74166667 -0.7375 -0.73333333 -0.72916667 -0.725 -0.72083333 -0.71666667 -0.7125 -0.70833333 -0.70416667 -0.7 -0.69583333 -0.69166667 -0.6875 -0.68333333 -0.67916667 -0.675 -0.67083333 -0.66666667 -0.6625 -0.65833333 -0.65416667 -0.65 -0.64583333 -0.64166667 -0.6375 -0.63333333 -0.62916667 -0.625 -0.62083333 -0.61666667 -0.6125 -0.60833333 -0.60416667 -0.6 -0.59583333 -0.59166667 -0.5875 -0.58333333 -0.57916667 -0.575 -0.57083333 -0.56666667 -0.5625 -0.55833333 -0.55416667 -0.55 -0.54583333 -0.54166667 -0.5375 -0.53333333 -0.52916667 -0.525 -0.52083333 -0.51666667 -0.5125 -0.50833333 -0.50416667 -0.5 -0.49583333 -0.49166667 -0.4875 -0.48333333 -0.47916667 -0.475 -0.47083333 -0.46666667 -0.4625 -0.45833333 -0.45416667 -0.45 -0.44583333 -0.44166667 -0.4375 -0.43333333 -0.42916667 -0.425 -0.42083333 -0.41666667 -0.4125 -0.40833333 -0.40416667 -0.4 -0.39583333 -0.39166667 -0.3875 -0.38333333 -0.37916667 -0.375 -0.37083333 -0.36666667 -0.3625 -0.35833333 -0.35416667 -0.35 -0.34583333 -0.34166667 -0.3375 -0.33333333 -0.32916667 -0.325 -0.32083333 -0.31666667 -0.3125 -0.30833333 -0.30416667 -0.3 -0.29583333 -0.29166667 -0.2875 -0.28333333 -0.27916667 -0.275 -0.27083333 -0.26666667 -0.2625 -0.25833333 -0.25416667 -0.25 -0.24583333 -0.24166667 -0.2375 -0.23333333 -0.22916667 -0.225 -0.22083333 -0.21666667 -0.2125 -0.20833333 -0.20416667 -0.2 -0.19583333 -0.19166667 -0.1875 -0.18333333 -0.17916667 -0.175 -0.17083333 -0.16666667 -0.1625 -0.15833333 -0.15416667 -0.15 -0.14583333 -0.14166667 -0.1375 -0.13333333 -0.12916667 -0.125 -0.12083333 -0.11666667 -0.1125 -0.10833333 -0.10416667 -0.1 -0.09583333 -0.09166667 -0.0875 -0.08333333 -0.07916667 -0.075 -0.07083333 -0.06666667 -0.0625 -0.05833333 -0.05416667 -0.05 -0.04583333 -0.04166667 -0.0375 -0.03333333 -0.02916667 -0.025 -0.02083333 -0.01666667 -0.0125 -0.00833333 -0.00416667 0 0 0 0 0 0
  line L11 (-28.5878, 17.6346) -> (-28.587, 17.6345)
  line L12 (-28.587, 17.6345) -> (-28.2972, 17.5824)
  arc A6 (-28.2972, 17.5824) -> (-28.4828, 16.4106) centre (0, 12.5) ccw
  line L13 (-28.4828, 16.4106) -> (-28.7745, 16.4507)
  line L14 (-28.7745, 16.4507) -> (-28.7753, 16.4508)
  spline S6 degree 5 poles (-28.7753, 16.4508) (-28.7754, 16.4508) (-28.7756, 16.4508) (-28.7759, 16.4509) (-28.7764, 16.4509) (-28.7772, 16.451) (-28.778, 16.4511) (-28.779, 16.4512) (-28.7801, 16.4514) (-28.7813, 16.4515) (-28.7826, 16.4517) (-28.784, 16.4518) (-28.7855, 16.452) (-28.7871, 16.4522) (-28.7889, 16.4523) (-28.7907, 16.4525) (-28.7926, 16.4527) (-28.7946, 16.4529) (-28.7968, 16.4531) (-28.799, 16.4534) (-28.8013, 16.4536) (-28.8037, 16.4538) (-28.8063, 16.454) (-28.8089, 16.4543) (-28.8116, 16.4545) (-28.8144, 16.4547) (-28.8172, 16.455) (-28.8202, 16.4552) (-28.8233, 16.4555) (-28.8264, 16.4557) (-28.8297, 16.4559) (-28.833, 16.4562) (-28.8364, 16.4564) (-28.8399, 16.4567) (-28.8435, 16.4569) (-28.8472, 16.4572) (-28.8509, 16.4574) (-28.8547, 16.4577) (-28.8586, 16.4579) (-28.8626, 16.4581) (-28.8667, 16.4584) (-28.8709, 16.4586) (-28.8751, 16.4588) (-28.8794, 16.459) (-28.8838, 16.4593) (-28.8882, 16.4595) (-28.8928, 16.4597) (-28.8974, 16.4599) (-28.9021, 16.4601) (-28.9068, 16.4603) (-28.9117, 16.4605) (-28.9166, 16.4607) (-28.9215, 16.4609) (-28.9266, 16.461) (-28.9317, 16.4612) (-28.9369, 16.4614) (-28.9422, 16.4615) (-28.9475, 16.4617) (-28.9529, 16.4618) (-28.9584, 16.462) (-28.9639, 16.4621) (-28.9695, 16.4622) (-28.9752, 16.4623) (-28.9809, 16.4624) (-28.9867, 16.4625) (-28.9926, 16.4626) (-28.9985, 16.4627) (-29.0045, 16.4627) (-29.0106, 16.4628) (-29.0167, 16.4629) (-29.0229, 16.4629) (-29.0291, 16.4629) (-29.0355, 16.4629) (-29.0418, 16.463) (-29.0483, 16.463) (-29.0548, 16.4629) (-29.0613, 16.4629) (-29.068, 16.4629) (-29.0746, 16.4628) (-29.0814, 16.4628) (-29.0882, 16.4627) (-29.095, 16.4626) (-29.1019, 16.4626) (-29.1089, 16.4625) (-29.1159, 16.4623) (-29.123, 16.4622) (-29.1302, 16.4621) (-29.1374, 16.4619) (-29.1446, 16.4618) (-29.1519, 16.4616) (-29.1593, 16.4614) (-29.1667, 16.4612) (-29.1742, 16.461) (-29.1817, 16.4607) (-29.1893, 16.4605) (-29.197, 16.4603) (-29.2047, 16.46) (-29.2124, 16.4597) (-29.2202, 16.4594) (-29.2281, 16.4591) (-29.236, 16.4588) (-29.2439, 16.4584) (-29.2519, 16.4581) (-29.26, 16.4577) (-29.2681, 16.4573) (-29.2763, 16.4569) (-29.2845, 16.4565) (-29.2927, 16.4561) (-29.301, 16.4556) (-29.3094, 16.4552) (-29.3178, 16.4547) (-29.3263, 16.4542) (-29.3348, 16.4537) (-29.3433, 16.4532) (-29.3519, 16.4526) (-29.3606, 16.4521) (-29.3693, 16.4515) (-29.378, 16.4509) (-29.3868, 16.4503) (-29.3957, 16.4497) (-29.4045, 16.4491) (-29.4135, 16.4484) (-29.4225, 16.4478) (-29.4315, 16.4471) (-29.4406, 16.4464) (-29.4497, 16.4457) (-29.4588, 16.4449) (-29.468, 16.4442) (-29.4773, 16.4434) (-29.4866, 16.4426) (-29.4959, 16.4418) (-29.5053, 16.441) (-29.5147, 16.4402) (-29.5242, 16.4393) (-29.5337, 16.4384) (-29.5433, 16.4375) (-29.5529, 16.4366) (-29.5625, 16.4357) (-29.5722, 16.4348) (-29.5819, 16.4338) (-29.5917, 16.4328) (-29.6015, 16.4318) (-29.6113, 16.4308) (-29.6212, 16.4297) (-29.6312, 16.4287) (-29.6411, 16.4276) (-29.6512, 16.4265) (-29.6612, 16.4254) (-29.6713, 16.4243) (-29.6814, 16.4231) (-29.6916, 16.422) (-29.7018, 16.4208) (-29.7121, 16.4196) (-29.7224, 16.4183) (-29.7327, 16.4171) (-29.7431, 16.4158) (-29.7535, 16.4145) (-29.764, 16.4132) (-29.7744, 16.4119) (-29.785, 16.4106) (-29.7955, 16.4092) (-29.8061, 16.4078) (-29.8168, 16.4064) (-29.8274, 16.405) (-29.8382, 16.4035) (-29.8489, 16.4021) (-29.8597, 16.4006) (-29.8705, 16.3991) (-29.8814, 16.3976) (-29.8923, 16.396) (-29.9032, 16.3945) (-29.9142, 16.3929) (-29.9252, 16.3913) (-29.9362, 16.3896) (-29.9473, 16.388) (-29.9584, 16.3863) (-29.9696, 16.3846) (-29.9807, 16.3829) (-29.992, 16.3812) (-30.0032, 16.3795) (-30.0145, 16.3777) (-30.0258, 16.3759) (-30.0372, 16.3741) (-30.0486, 16.3722) (-30.06, 16.3704) (-30.0714, 16.3685) (-30.0829, 16.3666) (-30.0944, 16.3647) (-30.106, 16.3628) (-30.1176, 16.3608) (-30.1292, 16.3588) (-30.1409, 16.3568) (-30.1525, 16.3548) (-30.1643, 16.3527) (-30.176, 16.3507) (-30.1878, 16.3486) (-30.1996, 16.3464) (-30.2115, 16.3443) (-30.2233, 16.3422) (-30.2353, 16.34) (-30.2472, 16.3378) (-30.2592, 16.3356) (-30.2712, 16.3333) (-30.2832, 16.331) (-30.2953, 16.3288) (-30.3074, 16.3264) (-30.3195, 16.3241) (-30.3317, 16.3217) (-30.3439, 16.3194) (-30.3561, 16.317) (-30.3683, 16.3145) (-30.3806, 16.3121) (-30.3929, 16.3096) (-30.4053, 16.3071) (-30.4176, 16.3046) (-30.43, 16.3021) (-30.4424, 16.2995) (-30.4549, 16.297) (-30.4674, 16.2943) (-30.4799, 16.2917) (-30.4924, 16.2891) (-30.505, 16.2864) (-30.5176, 16.2837) (-30.5302, 16.281) (-30.5429, 16.2782) (-30.5556, 16.2755) (-30.5683, 16.2727) (-30.581, 16.2699) (-30.5938, 16.267) (-30.6066, 16.2642) (-30.6194, 16.2613) (-30.6323, 16.2584) (-30.6451, 16.2555) (-30.658, 16.2525) (-30.671, 16.2496) (-30.6839, 16.2466) (-30.6969, 16.2435) (-30.7099, 16.2405) (-30.723, 16.2374) (-30.736, 16.2343) (-30.7491, 16.2312) (-30.7596, 16.2287) (-30.7675, 16.2268) (-30.7728, 16.2256) (-30.7754, 16.2249) knots 0 0 0 0 0 0 0.00416667 0.00833333 0.0125 0.01666667 0.02083333 0.025 0.02916667 0.03333333 0.0375 0.04166667 0.04583333 0.05 0.05416667 0.05833333 0.0625 0.06666667 0.07083333 0.075 0.07916667 0.08333333 0.0875 0.09166667 0.09583333 0.1 0.10416667 0.10833333 0.1125 0.11666667 0.12083333 0.125 0.12916667 0.13333333 0.1375 0.14166667 0.14583333 0.15 0.15416667 0.15833333 0.1625 0.16666667 0.17083333 0.175 0.17916667 0.18333333 0.1875 0.19166667 0.19583333 0.2 0.20416667 0.20833333 0.2125 0.21666667 0.22083333 0.225 0.22916667 0.23333333 0.2375 0.24166667 0.24583333 0.25 0.25416667 0.25833333 0.2625 0.26666667 0.27083333 0.275 0.27916667 0.28333333 0.2875 0.29166667 0.29583333 0.3 0.30416667 0.30833333 0.3125 0.31666667 0.32083333 0.325 0.32916667 0.33333333 0.3375 0.34166667 0.34583333 0.35 0.35416667 0.35833333 0.3625 0.36666667 0.37083333 0.375 0.37916667 0.38333333 0.3875 0.39166667 0.39583333 0.4 0.40416667 0.40833333 0.4125 0.41666667 0.42083333 0.425 0.42916667 0.43333333 0.4375 0.44166667 0.44583333 0.45 0.45416667 0.45833333 0.4625 0.46666667 0.47083333 0.475 0.47916667 0.48333333 0.4875 0.49166667 0.49583333 0.5 0.50416667 0.50833333 0.5125 0.51666667 0.52083333 0.525 0.52916667 0.53333333 0.5375 0.54166667 0.54583333 0.55 0.55416667 0.55833333 0.5625 0.56666667 0.57083333 0.575 0.57916667 0.58333333 0.5875 0.59166667 0.59583333 0.6 0.60416667 0.60833333 0.6125 0.61666667 0.62083333 0.625 0.62916667 0.63333333 0.6375 0.64166667 0.64583333 0.65 0.65416667 0.65833333 0.6625 0.66666667 0.67083333 0.675 0.67916667 0.68333333 0.6875 0.69166667 0.69583333 0.7 0.70416667 0.70833333 0.7125 0.71666667 0.72083333 0.725 0.72916667 0.73333333 0.7375 0.74166667 0.74583333 0.75 0.75416667 0.75833333 0.7625 0.76666667 0.77083333 0.775 0.77916667 0.78333333 0.7875 0.79166667 0.79583333 0.8 0.80416667 0.80833333 0.8125 0.81666667 0.82083333 0.825 0.82916667 0.83333333 0.8375 0.84166667 0.84583333 0.85 0.85416667 0.85833333 0.8625 0.86666667 0.87083333 0.875 0.87916667 0.88333333 0.8875 0.89166667 0.89583333 0.9 0.90416667 0.90833333 0.9125 0.91666667 0.92083333 0.925 0.92916667 0.93333333 0.9375 0.94166667 0.94583333 0.95 0.95416667 0.95833333 0.9625 0.96666667 0.97083333 0.975 0.97916667 0.98333333 0.9875 0.99166667 0.99583333 1 1 1 1 1 1
  arc A7 (-30.7754, 16.2249) -> (-30.8773, 15.255) centre (0, 12.5) ccw
  spline S7 degree 5 poles (-30.8773, 15.255) (-30.8749, 15.2539) (-30.87, 15.2515) (-30.8627, 15.248) (-30.853, 15.2434) (-30.8408, 15.2376) (-30.8287, 15.2319) (-30.8165, 15.2262) (-30.8044, 15.2205) (-30.7924, 15.2149) (-30.7803, 15.2092) (-30.7683, 15.2036) (-30.7563, 15.1981) (-30.7443, 15.1925) (-30.7323, 15.187) (-30.7204, 15.1815) (-30.7085, 15.1761) (-30.6966, 15.1707) (-30.6847, 15.1653) (-30.6728, 15.1599) (-30.661, 15.1545) (-30.6492, 15.1492) (-30.6374, 15.1439) (-30.6256, 15.1387) (-30.6139, 15.1335) (-30.6022, 15.1283) (-30.5905, 15.1231) (-30.5788, 15.1179) (-30.5672, 15.1128) (-30.5555, 15.1077) (-30.5439, 15.1027) (-30.5324, 15.0977) (-30.5208, 15.0927) (-30.5093, 15.0877) (-30.4978, 15.0827) (-30.4863, 15.0778) (-30.4749, 15.0729) (-30.4634, 15.0681) (-30.452, 15.0632) (-30.4407, 15.0584) (-30.4293, 15.0537) (-30.418, 15.0489) (-30.4067, 15.0442) (-30.3954, 15.0395) (-30.3841, 15.0348) (-30.3729, 15.0302) (-30.3617, 15.0256) (-30.3506, 15.021) (-30.3394, 15.0165) (-30.3283, 15.0119) (-30.3172, 15.0074) (-30.3061, 15.003) (-30.2951, 14.9985) (-30.2841, 14.9941) (-30.2731, 14.9897) (-30.2621, 14.9854) (-30.2512, 14.981) (-30.2403, 14.9767) (-30.2294, 14.9725) (-30.2186, 14.9682) (-30.2078, 14.964) (-30.197, 14.9598) (-30.1862, 14.9557) (-30.1755, 14.9515) (-30.1648, 14.9474) (-30.1541, 14.9433) (-30.1435, 14.9393) (-30.1329, 14.9353) (-30.1223, 14.9313) (-30.1118, 14.9273) (-30.1012, 14.9234) (-30.0907, 14.9194) (-30.0803, 14.9156) (-30.0699, 14.9117) (-30.0595, 14.9079) (-30.0491, 14.9041) (-30.0388, 14.9003) (-30.0284, 14.8965) (-30.0182, 14.8928) (-30.0079, 14.8891) (-29.9977, 14.8855) (-29.9875, 14.8818) (-29.9774, 14.8782) (-29.9673, 14.8746) (-29.9572, 14.8711) (-29.9471, 14.8675) (-29.9371, 14.864) (-29.9271, 14.8606) (-29.9172, 14.8571) (-29.9073, 14.8537) (-29.8974, 14.8503) (-29.8875, 14.8469) (-29.8777, 14.8436) (-29.868, 14.8403) (-29.8582, 14.837) (-29.8485, 14.8337) (-29.8388, 14.8305) (-29.8292, 14.8273) (-29.8196, 14.8241) (-29.81, 14.821) (-29.8005, 14.8178) (-29.791, 14.8147) (-29.7815, 14.8117) (-29.7721, 14.8086) (-29.7627, 14.8056) (-29.7534, 14.8026) (-29.7441, 14.7996) (-29.7348, 14.7967) (-29.7255, 14.7938) (-29.7163, 14.7909) (-29.7072, 14.788) (-29.6981, 14.7852) (-29.689, 14.7824) (-29.6799, 14.7796) (-29.6709, 14.7769) (-29.6619, 14.7741) (-29.653, 14.7714) (-29.6441, 14.7688) (-29.6353, 14.7661) (-29.6265, 14.7635) (-29.6177, 14.7609) (-29.609, 14.7583) (-29.6003, 14.7558) (-29.5917, 14.7533) (-29.583, 14.7508) (-29.5745, 14.7483) (-29.566, 14.7458) (-29.5575, 14.7434) (-29.5491, 14.741) (-29.5407, 14.7387) (-29.5323, 14.7363) (-29.524, 14.734) (-29.5158, 14.7317) (-29.5075, 14.7295) (-29.4994, 14.7272) (-29.4912, 14.725) (-29.4832, 14.7228) (-29.4751, 14.7207) (-29.4671, 14.7185) (-29.4592, 14.7164) (-29.4513, 14.7143) (-29.4434, 14.7123) (-29.4356, 14.7102) (-29.4279, 14.7082) (-29.4202, 14.7062) (-29.4125, 14.7043) (-29.4049, 14.7023) (-29.3973, 14.7004) (-29.3898, 14.6985) (-29.3823, 14.6967) (-29.3749, 14.6948) (-29.3675, 14.693) (-29.3602, 14.6912) (-29.3529, 14.6895) (-29.3457, 14.6877) (-29.3386, 14.686) (-29.3314, 14.6843) (-29.3244, 14.6827) (-29.3174, 14.681) (-29.3104, 14.6794) (-29.3035, 14.6778) (-29.2967, 14.6762) (-29.2899, 14.6747) (-29.2831, 14.6731) (-29.2764, 14.6716) (-29.2698, 14.6702) (-29.2632, 14.6687) (-29.2567, 14.6673) (-29.2502, 14.6659) (-29.2438, 14.6645) (-29.2374, 14.6631) (-29.2311, 14.6618) (-29.2249, 14.6605) (-29.2187, 14.6592) (-29.2126, 14.6579) (-29.2065, 14.6567) (-29.2005, 14.6554) (-29.1946, 14.6542) (-29.1887, 14.653) (-29.1829, 14.6519) (-29.1771, 14.6507) (-29.1714, 14.6496) (-29.1658, 14.6485) (-29.1602, 14.6475) (-29.1547, 14.6464) (-29.1493, 14.6454) (-29.1439, 14.6444) (-29.1386, 14.6434) (-29.1334, 14.6424) (-29.1282, 14.6415) (-29.1231, 14.6406) (-29.118, 14.6397) (-29.1131, 14.6388) (-29.1081, 14.638) (-29.1033, 14.6371) (-29.0985, 14.6363) (-29.0938, 14.6355) (-29.0892, 14.6347) (-29.0847, 14.634) (-29.0802, 14.6332) (-29.0758, 14.6325) (-29.0714, 14.6318) (-29.0672, 14.6312) (-29.063, 14.6305) (-29.0589, 14.6299) (-29.0549, 14.6292) (-29.0509, 14.6286) (-29.047, 14.6281) (-29.0432, 14.6275) (-29.0395, 14.627) (-29.0359, 14.6264) (-29.0323, 14.6259) (-29.0289, 14.6254) (-29.0255, 14.625) (-29.0222, 14.6245) (-29.0189, 14.6241) (-29.0158, 14.6237) (-29.0128, 14.6233) (-29.0098, 14.6229) (-29.0069, 14.6225) (-29.0041, 14.6222) (-29.0015, 14.6219) (-28.9989, 14.6215) (-28.9963, 14.6212) (-28.9939, 14.621) (-28.9916, 14.6207) (-28.9894, 14.6204) (-28.9873, 14.6202) (-28.9852, 14.62) (-28.9833, 14.6198) (-28.9815, 14.6196) (-28.9798, 14.6194) (-28.9781, 14.6192) (-28.9766, 14.6191) (-28.9752, 14.6189) (-28.9739, 14.6188) (-28.9727, 14.6187) (-28.9716, 14.6186) (-28.9706, 14.6185) (-28.9698, 14.6184) (-28.969, 14.6184) (-28.9685, 14.6183) (-28.9682, 14.6183) (-28.968, 14.6183) (-28.9679, 14.6183) knots -1 -1 -1 -1 -1 -1 -0.99583333 -0.99166667 -0.9875 -0.98333333 -0.97916667 -0.975 -0.97083333 -0.96666667 -0.9625 -0.95833333 -0.95416667 -0.95 -0.94583333 -0.94166667 -0.9375 -0.93333333 -0.92916667 -0.925 -0.92083333 -0.91666667 -0.9125 -0.90833333 -0.90416667 -0.9 -0.89583333 -0.89166667 -0.8875 -0.88333333 -0.87916667 -0.875 -0.87083333 -0.86666667 -0.8625 -0.85833333 -0.85416667 -0.85 -0.84583333 -0.84166667 -0.8375 -0.83333333 -0.82916667 -0.825 -0.82083333 -0.81666667 -0.8125 -0.80833333 -0.80416667 -0.8 -0.79583333 -0.79166667 -0.7875 -0.78333333 -0.77916667 -0.775 -0.77083333 -0.76666667 -0.7625 -0.75833333 -0.75416667 -0.75 -0.74583333 -0.74166667 -0.7375 -0.73333333 -0.72916667 -0.725 -0.72083333 -0.71666667 -0.7125 -0.70833333 -0.70416667 -0.7 -0.69583333 -0.69166667 -0.6875 -0.68333333 -0.67916667 -0.675 -0.67083333 -0.66666667 -0.6625 -0.65833333 -0.65416667 -0.65 -0.64583333 -0.64166667 -0.6375 -0.63333333 -0.62916667 -0.625 -0.62083333 -0.61666667 -0.6125 -0.60833333 -0.60416667 -0.6 -0.59583333 -0.59166667 -0.5875 -0.58333333 -0.57916667 -0.575 -0.57083333 -0.56666667 -0.5625 -0.55833333 -0.55416667 -0.55 -0.54583333 -0.54166667 -0.5375 -0.53333333 -0.52916667 -0.525 -0.52083333 -0.51666667 -0.5125 -0.50833333 -0.50416667 -0.5 -0.49583333 -0.49166667 -0.4875 -0.48333333 -0.47916667 -0.475 -0.47083333 -0.46666667 -0.4625 -0.45833333 -0.45416667 -0.45 -0.44583333 -0.44166667 -0.4375 -0.43333333 -0.42916667 -0.425 -0.42083333 -0.41666667 -0.4125 -0.40833333 -0.40416667 -0.4 -0.39583333 -0.39166667 -0.3875 -0.38333333 -0.37916667 -0.375 -0.37083333 -0.36666667 -0.3625 -0.35833333 -0.35416667 -0.35 -0.34583333 -0.34166667 -0.3375 -0.33333333 -0.32916667 -0.325 -0.32083333 -0.31666667 -0.3125 -0.30833333 -0.30416667 -0.3 -0.29583333 -0.29166667 -0.2875 -0.28333333 -0.27916667 -0.275 -0.27083333 -0.26666667 -0.2625 -0.25833333 -0.25416667 -0.25 -0.24583333 -0.24166667 -0.2375 -0.23333333 -0.22916667 -0.225 -0.22083333 -0.21666667 -0.2125 -0.20833333 -0.20416667 -0.2 -0.19583333 -0.19166667 -0.1875 -0.18333333 -0.17916667 -0.175 -0.17083333 -0.16666667 -0.1625 -0.15833333 -0.15416667 -0.15 -0.14583333 -0.14166667 -0.1375 -0.13333333 -0.12916667 -0.125 -0.12083333 -0.11666667 -0.1125 -0.10833333 -0.10416667 -0.1 -0.09583333 -0.09166667 -0.0875 -0.08333333 -0.07916667 -0.075 -0.07083333 -0.06666667 -0.0625 -0.05833333 -0.05416667 -0.05 -0.04583333 -0.04166667 -0.0375 -0.03333333 -0.02916667 -0.025 -0.02083333 -0.01666667 -0.0125 -0.00833333 -0.00416667 0 0 0 0 0 0
  line L15 (-28.9679, 14.6183) -> (-28.9671, 14.6182)
  line L16 (-28.9671, 14.6182) -> (-28.6734, 14.5967)
  arc A8 (-28.6734, 14.5967) -> (-28.7355, 13.4119) centre (0, 12.5) ccw
  line L17 (-28.7355, 13.4119) -> (-29.0298, 13.4213)
  line L18 (-29.0298, 13.4213) -> (-29.0307, 13.4213)